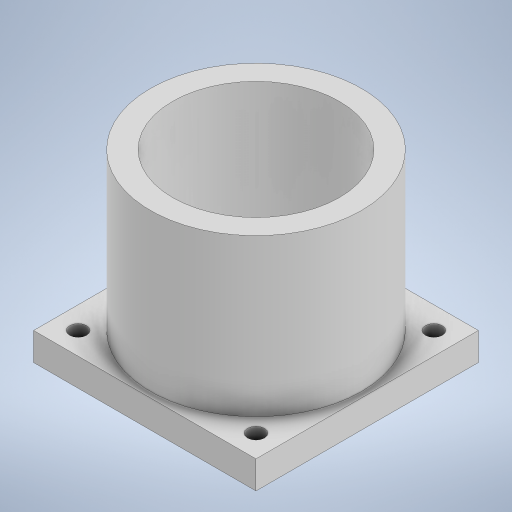
# Autodesk Inventor part: Cylinders
Saved by Autodesk Inventor 2023 (Build 270158000, 158)
## iProperties
Created: 2022-10-26
Part Number: Cylinders
Material: Generic
Document SubType Name: Modeling
Designer: tommy
Density: 1 g/cm^3
Appearance: Default
Author: tommy
Autodesk Inventor part; units mm, degrees
ref_plane "YZ Plane" through (0, 0, 0) normal (1, 0, 0) x (0, 1, 0)
ref_plane "XZ Plane" through (0, 0, 0) normal (0, 1, 0) x (-1, 0, 0)
ref_plane "XY Plane" through (0, 0, 0) normal (0, 0, 1) x (1, 0, 0)
sketch "Sketch1" plane through (0, 0, 0) normal (0, 1, 0) x (-1, 0, 0)
  circle A0 centre (0, 0) radius 19.05
  circle A1 centre (0, 0) radius 24.13
  line L0 (25.4, 25.4) -> (-25.4, 25.4)
  line L1 (-25.4, 25.4) -> (-25.4, -25.4)
  line L2 (-25.4, -25.4) -> (25.4, -25.4)
  line L3 (25.4, -25.4) -> (25.4, 25.4)
  line L4 (-25.4, -25.4) -> (-12.1092, -25.4) construction
  circle A2 centre (-20.32, -20.32) radius 1.9304
  circle A3 centre (-20.32, 20.32) radius 1.9304
  circle A4 centre (20.32, -20.32) radius 1.9304
  circle A5 centre (20.32, 20.32) radius 1.9304
  dimension "d10" = 50.8
  dimension "d11" = 50.8
  dimension "d20" = 3.8608
  dimension "d25" = 3.8608
  dimension "d26" = 3.8608
  dimension "d27" = 3.8608
  constraints: 10 end point, 6 centre point, 2 horizontal, 2 parallel, 1 coincident, 1 perpendicular
  measures "d10" distance of L0.start L0.end
  measures "d11" distance of L1.end L0.end
  measures "d20" diameter of A2
  measures "d25" diameter of A4
  measures "d26" diameter of A5
  measures "d27" diameter of A3
extrude "Extrusion1" add sketch "Sketch1" along normal blind 42.164 contours A1
extrude "Extrusion3" add sketch "Sketch1" along normal blind 6.35 contours A1 | L3 L2 L1 L0 | A2 | A3 | A4 | A5
extrude "Extrusion5" cut sketch "Sketch1" along normal blind 6.35 contours A2 | A3 | A4 | A5
body "Solid1"
